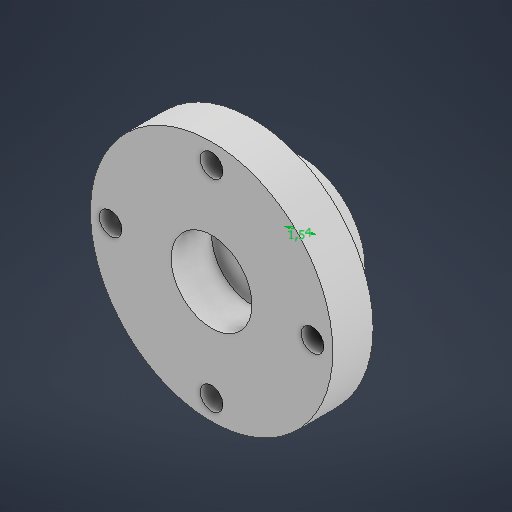
# Autodesk Inventor part: motor dişlisi
Saved by Autodesk Inventor 2026.1 (Build 301233020, 233B)
## iProperties
Created: 2026-04-08
Part Number: motor dişlisi
Material: Generic
Document SubType Name: Modeling
Designer: kadir
Density: 1 g/cm^3
Appearance: Default
Author: kadir
Autodesk Inventor part; units mm, degrees
ref_plane "YZ Plane" through (0, 0, 0) normal (1, 0, 0) x (0, 1, 0)
ref_plane "XZ Plane" through (0, 0, 0) normal (0, 1, 0) x (-1, 0, 0)
ref_plane "XY Plane" through (0, 0, 0) normal (0, 0, 1) x (1, 0, 0)
sketch "Sketch1" plane through (0, 0, 0) normal (0, 0, 1) x (1, 0, 0)
  circle A0 centre (0, 0) radius 2
  circle A1 centre (0, 0) radius 8
  dimension "d0" = 4
  dimension "d1" = 16
  constraints: 2 centre point, 2 coincident
  measures "d0" diameter of A0
  measures "d1" diameter of A1
extrude "Extrusion1" add sketch "Sketch1" along normal blind 6
sketch "Sketch2" plane through (0, 0, 6) normal (0, 0, 1) x (1, 0, 0)
  circle A0 centre (0, 0) radius 5
  circle A1 centre (0, 0) radius 15
  dimension "d4" = 10
  dimension "d5" = 30
  constraints: 2 centre point, 2 coincident
  measures "d4" diameter of A0
  measures "d5" diameter of A1
extrude "Extrusion2" add sketch "Sketch2" along normal blind 5
sketch "Sketch5" plane through (0, 0, 6) normal (0, 0, -1) x (-1, 0, 0)
  circle A0 centre (0, 12.5) radius 1.4
  circle A1 centre (-12.5, 0) radius 1.4
  circle A2 centre (0, -12.5) radius 1.4
  circle A3 centre (12.5, 0) radius 1.4
  point P0 (0, 0)
  dimension "d24" = 12.5
  dimension "d25" = 2.8
  dimension "d28" = 360
  constraints: 4 centre point, 1 vertical alignment, 9 other
  measures "d24" distance of point (0, 0) A0.centre
  measures "d25" diameter of A0
extrude "Extrusion5" cut sketch "Sketch5" against normal blind 10 contours A0 | A1 | A3
sketch "Sketch6" plane through (0, 0, 11) normal (0, 0, 1) x (1, 0, 0)
  circle A0 centre (0, -12.5) radius 1.4
  point P0 (0, 0)
  dimension "d42" = 2.8
  dimension "d43" = 12.5
  constraints: 1 centre point, 1 vertical alignment
  measures "d42" diameter of A0
  measures "d43" distance of A0.centre point (0, 0)
extrude "Extrusion6" cut sketch "Sketch6" against normal blind 10
sketch "Sketch9" plane through (0, 0, 0) normal (0, 0, -1) x (-1, 0, 0)
  line L0 (1.5, 2.0687) -> (1.5, -2.0687)
  circle A0 centre (0, 0) radius 2
  point P0 (1.5, 1.3229)
  point P1 (1.5, -1.3229)
  dimension "d46" = 4
  dimension "d47" = 1.5
  constraints: 2 end point, 1 centre point, 1 coincident, 1 vertical
  measures "d46" diameter of A0
  measures "d47" distance from line of point (0, 0) L0
extrude "Extrusion7" add sketch "Sketch9" against normal blind 6 contours A0 L0 picked at (1.7382, -0.2911)
sketch "Sketch11" plane through (0, 0, 0) normal (1, 0, 0) x (0, 1, 0)
  circle A0 centre (0, 3) radius 1
  line L0 (8, 0) -> (-8, 0) projected
  point P0 (0, 0)
  dimension "d50" = 2
  dimension "d51" = 3
  constraints: 1 centre point
  measures "d50" diameter of A0
  measures "d51" distance from line of L0 A0.centre
extrude "Extrusion8" cut sketch "Sketch11" against normal blind 10
sketch "Sketch12" plane through (0, 0, 6) normal (0, 0, -1) x (-1, 0, 0)
  point P0 (0, 0)
sketch "Sketch13" plane through (0, 0, 6) normal (0, 0, -1) x (-1, 0, 0)
  point P0 (0, 0)
body "Solid1"
